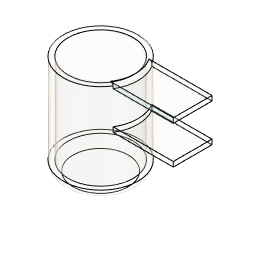
Desk Can Holder - 330ml v2 (Autodesk Fusion 360 design; units mm, degrees)
Autodesk Fusion 360 part; units mm, degrees
sketch "Sketch1" plane through (0, 0, 0) normal (0, 0, 1) x (1, 0, 0)
  circle A0 centre (51.0584, 63.823) radius 33.5
  circle A1 centre (51.0584, 63.823) radius 38.5
  dimension "d1" = 67
  dimension "d2" = 77
  constraint concentric A0 A1
  measures "d1" diameter of A0
  measures "d2" diameter of A1
extrude "Extrude1" add sketch "Sketch1" along normal blind 95 makes body 1
sketch "Sketch2" plane through (0, 0, 0) normal (0, 0, -1) x (1, 0, 0)
  circle A0 centre (51.0584, -63.823) radius 33.5
  circle A1 centre (51.0584, -63.823) radius 38.5
  circle A2 centre (51.0584, -63.823) radius 33.5
  constraint concentric A0 A2
extrude "Extrude2" add sketch "Sketch2" along normal blind 10 contours A0 A2 | A1 bodies 1
fillet "Fillet1" radius 10 1 edges at (15.1638, 77.7452, -10) on bodies 1
sketch "Sketch3" plane through (0, 0, 95) normal (0, 0, 1) x (-1, 0, 0)
  circle A0 centre (-51.0584, -63.823) radius 33.5
  circle A1 centre (-51.0584, -63.823) radius 38.5
  line L0 (-51.0584, -63.823) -> (-51.0584, -83.823)
  line L1 (-51.0584, -83.823) -> (-121.0584, -83.823)
  line L2 (-121.0584, -83.823) -> (-121.0584, -43.823)
  line L3 (-121.0584, -43.823) -> (-51.0584, -43.823)
  line L4 (-51.0584, -43.823) -> (-51.0584, -83.823)
  dimension "d9" = 20
  dimension "d10" = 70
  dimension "d11" = 40
  constraint coincident A0.centre A1.centre
  constraint vertical L0
  constraint horizontal L1
  constraint vertical L2
  constraint horizontal L3
  constraint vertical L4
  measures "d9" distance of A0.centre L0.end
  measures "d10" distance of L0.end L1.end
  measures "d11" distance of L0.end L3.end
extrude "Extrude3" add sketch "Sketch3" against normal blind 5 contours A1 L1 L2 L3 bodies 1
sketch "Sketch4" plane through (0, 43.823, 0) normal (0, -1, 0) x (1, 0, 0)
  line L0 (121.0584, 95) -> (83.956, 95)
  line L1 (83.956, 95) -> (83.956, 90)
  line L2 (83.956, 90) -> (121.0584, 90)
  line L3 (121.0584, 90) -> (121.0584, 95)
  line L4 (121.0584, 90) -> (121.0584, 55.9)
  line L5 (121.0584, 55.9) -> (82.9536, 55.9)
  line L6 (82.9536, 55.9) -> (192.9536, 55.9)
  line L7 (192.9536, 55.9) -> (192.9536, 50.9)
  line L8 (192.9536, 50.9) -> (82.9536, 50.9)
  line L9 (82.9536, 50.9) -> (82.9536, 55.9)
  dimension "d14" = 34.1
  dimension "d15" = 110
  dimension "d16" = 5
  constraint coincident L2.end L3.start
  constraint perpendicular L2 L4
  constraint perpendicular L4 L5
  constraint horizontal L6
  constraint vertical L7
  constraint horizontal L8
  constraint vertical L9
  measures "d14" distance of L2.end L4.end
  measures "d15" distance of L5.end L6.end
  measures "d16" distance of L5.end L8.end
extrude "Extrude4" add sketch "Sketch4" against normal blind 40 contours L5 L6 L7 L8 L9 bodies 1
delete_face "DeleteFace1" 1 faces at (82.9536, 67.2379, 54.2333) on bodies 1
fillet "Fillet2" radius 2.5 1 edges at (19.8255, 75.9372, 95) on bodies 1
fillet "Fillet3" radius 2.5 1 edges at (12.5584, 63.823, 95) on bodies 1
move_body "Move1" bodies 1 to x (1, 0, 0) y (0, 1, 0) z (0, 0, 1) at (0, 0, 10)
extrude "Extrude5" add 1 faces at (121.0584, 70.4897, 101.6667) along direction (1, 0, 0) blind 25 on bodies 1 bodies 1
sketch "Sketch5" plane through (0, 43.823, 0) normal (0, -1, 0) x (1, 0, 0)
  line L0 (146.0584, 105) -> (80.9917, 105)
  spline S0 degree 3 poles (80.9917, 105) (81.3818, 105) (81.8432, 104.9204) (82.5386, 104.6595) (82.9032, 104.4448) (83.3993, 103.9945) (83.6282, 103.6902) (83.8798, 103.1348) (83.956, 102.7924) (83.956, 102.5) knots 1.229891 1.229891 1.229891 1.229891 1.346936 1.346936 1.452717 1.452717 1.547922 1.547922 1.635629 1.635629 1.635629 1.635629
  line L1 (83.956, 102.5) -> (83.956, 100)
  line L2 (83.956, 100) -> (146.0584, 100)
  line L3 (146.0584, 100) -> (146.0584, 105)
split "Split1" by plane through (146.0584, 83.823, 105) normal (1, 0, 0) bodies 1 makes body 2 at (177.3218, 70.4897, 60.9)
delete_body "RemoveBody1" bodies 2
